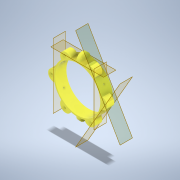
# Autodesk Inventor part: Connector
Saved by Autodesk Inventor 2021.2 (Build 252289000, 289)
## iProperties
Created: 2021-03-12
Part Number: Connector
Material: Generic
Document SubType Name: Modeling
Designer: Ryan
Density: 1 g/cm^3
Appearance: Smooth - Yellow
Author: Ryan
Autodesk Inventor part; units mm, degrees
ref_plane "XY Plane" through (0, 0, 0) normal (0, 0, 1) x (1, 0, 0)
sketch "Sketch1" plane through (0, 0, 0) normal (0, 0, 1) x (1, 0, 0)
  circle A0 centre (0, 0) radius 50.8
  circle A1 centre (0, 0) radius 53.975
  dimension "d0" = 101.6
  dimension "d1" = 107.95
  constraints: 2 centre point, 2 coincident
  measures "d0" diameter of A0
  measures "d1" diameter of A1
extrude "Extrusion1" add sketch "Sketch1" along normal blind 25.4
ref_plane "Work Plane1" through (38.1, 0, 0) normal (1, 0, 0) x (0, 1, 0)
ref_plane "Work Plane2" through (0, 53.975, 0) normal (0, 1, 0) x (-1, 0, 0)
sketch "Sketch3" plane through (0, 53.975, 0) normal (0, 1, 0) x (-1, 0, 0)
  line L0 (53.975, 0) -> (-53.975, 0) projected
  line L1 (3.175, 25.4) -> (-3.175, 25.4)
  line L2 (-3.175, 25.4) -> (-3.175, 0)
  line L3 (-3.175, 0) -> (3.175, 0)
  line L4 (3.175, 0) -> (3.175, 25.4)
  line L5 (3.175, 25.4) -> (-3.175, 0) construction
  line L6 (-3.175, 25.4) -> (3.175, 0) construction
  line L7 (53.975, 25.4) -> (-53.975, 25.4) projected
  point P0 (0, 0)
  point P1 (0, 12.7)
  point P2 (3.175, 0)
  dimension "d11" = 6.35
  dimension "d12" = 0
  constraints: 12 end point, 2 midpoint, 2 parallel, 1 horizontal, 1 perpendicular, 1 point on line
  measures "d11" distance of L3.end L2.end
  measures "d12" distance between parallel lines of L7 L1
extrude "Extrusion3" add sketch "Sketch3" along normal blind 12.7
fillet "Fillet1" radius 12.7 2 edges at (0, 66.675, 25.4) (0, 66.675, 0)
sketch "Sketch4" plane through (3.175, 53.975, 25.4) normal (1, 0, 0) x (0, 0, -1)
  circle A0 centre (6.35, 5.08) radius 1.5875
  line L0 (-5.08, 0) -> (30.48, 0) projected
  line L1 (0, 0) -> (0, -107.95) projected
  circle A1 centre (19.05, 5.08) radius 1.5875
  line L2 (25.4, 0) -> (25.4, -107.95) projected
  point P0 (25.4, -53.975)
  dimension "d16" = 3.175
  dimension "d17" = 5.08
  dimension "d40" = 6.35
  dimension "d41" = 3.175
  dimension "d42" = 6.35
  dimension "d43" = 5.08
  constraints: 2 centre point
  measures "d16" diameter of A0
  measures "d17" distance from line of L0 A0.centre
  measures "d40" horizontal distance of A0.centre L1.start
  measures "d41" diameter of A1
  measures "d42" horizontal distance of L2.start A1.centre
  measures "d43" distance from line of L0 A1.centre
extrude "Extrusion4" cut sketch "Sketch4" against normal blind 12.7
pattern_circular "Circular Pattern2" count 2 over 360 about axis through (0, 0, 0) along (0, 0, 1) of "Extrusion4", "Fillet1", "Extrusion3"
ref_plane "Work Plane3" through (-53.975, 0, 0) normal (1, 0, 0) x (0, 1, 0)
sketch "Sketch5" plane through (-53.975, 0, 0) normal (1, 0, 0) x (0, 1, 0)
  line L0 (-12.7, 9.525) -> (12.7, 9.525)
  line L1 (12.7, 9.525) -> (12.7, 15.875)
  line L2 (12.7, 15.875) -> (-12.7, 15.875)
  line L3 (-12.7, 15.875) -> (-12.7, 9.525)
  line L4 (-12.7, 9.525) -> (12.7, 15.875) construction
  line L5 (12.7, 9.525) -> (-12.7, 15.875) construction
  line L6 (53.975, 25.4) -> (-53.975, 25.4) projected
  line L7 (12.7, 15.875) -> (-12.7, 15.875)
  line L8 (-12.7, 15.875) -> (-12.7, 25.4)
  line L9 (-12.7, 25.4) -> (12.7, 25.4)
  line L10 (12.7, 25.4) -> (12.7, 15.875)
  point P0 (0, 0)
  point P1 (0, 12.7)
  point P2 (12.7, 25.4)
  dimension "d24" = 25.4
  dimension "d25" = 6.35
  dimension "d26" = 12.7
  dimension "d27" = 0
  constraints: 20 end point, 4 parallel, 2 horizontal, 2 midpoint, 2 perpendicular, 1 point on line
  measures "d24" distance of L2.end L1.end
  measures "d25" distance of L1.end L0.end
  measures "d26" distance of point (0, 12.7) point (0, 0)
  measures "d27" horizontal distance of point (0, 12.7) point (0, 0)
extrude "Extrusion8" add sketch "Sketch5" along normal blind 2.54
sketch "Sketch8" plane through (-53.975, 0, 0) normal (-1, 0, 0) x (0, 0, 1)
  line L0 (9.525, 0) -> (9.525, -12.7) projected
  line L1 (9.525, 12.7) -> (25.4, 12.7) projected
  line L2 (9.525, -12.7) -> (25.4, -12.7)
  line L3 (25.4, -12.7) -> (25.4, 12.7)
  line L4 (25.4, 12.7) -> (9.525, 12.7)
  line L5 (9.525, 12.7) -> (9.525, -12.7)
  point P0 (0, 0)
  constraints: 8 end point, 2 parallel, 1 horizontal, 1 perpendicular
extrude "Extrusion9" add sketch "Sketch8" along normal blind 12.7
fillet "Fillet3" radius 12.7 2 edges at (-66.675, 12.7, 17.4625) (-66.675, -12.7, 17.4625)
sketch "Sketch9" plane through (0, 0, 9.525) normal (0, 0, -1) x (-1, 0, 0)
  circle A0 centre (59.055, 0) radius 3.175
  line L0 (53.975, -93.345) -> (53.975, 93.345) projected
  point P0 (0, 0)
  dimension "d54" = 5.08
  dimension "d55" = 6.35
  constraints: 1 centre point
  measures "d54" distance from line of L0 A0.centre
  measures "d55" diameter of A0
extrude "Extrusion10" cut sketch "Sketch9" against normal through all
pattern_circular "Circular Pattern4" count 6 over 360 about axis through (0, 0, 0) along (0, 0, 1) of "Extrusion8", "Extrusion9", "Fillet3", "Extrusion10"
sketch "Sketch10" plane through (0, 53.975, 0) normal (0, 1, 0) x (-1, 0, 0)
  line L0 (3.175, 25.4) -> (3.175, 0) projected
  line L1 (-3.175, 0) -> (-3.175, 25.4) projected
  line L2 (3.175, 0) -> (-3.175, 0)
  line L3 (-3.175, 0) -> (-3.175, 25.4)
  line L4 (-3.175, 25.4) -> (3.175, 25.4)
  line L5 (3.175, 25.4) -> (3.175, 0)
  point P0 (0, 0)
  constraints: 8 end point, 2 parallel, 1 horizontal, 1 perpendicular
extrude "Extrusion11" add sketch "Sketch10" against normal blind 2.54
mirror "Mirror1" about plane through (0, 0, 0) normal (0, 1, 0) of "Extrusion11"
ref_plane "Work Plane4" through (46.7437, -26.9875, 0) normal (0.8660254, -0.5, 0) x (0.5, 0.8660254, 0)
sketch "Sketch11" plane through (46.7437, -26.9875, 0) normal (0.8660254, -0.5, 0) x (0.5, 0.8660254, 0)
  line L0 (12.5159, 12.7) -> (5.3749, 12.7)
  line L1 (53.975, 0) -> (-45.0753, 0) projected
  circle A0 centre (0, 12.7) radius 1.5875
  point P0 (0, 0)
  point P1 (48.2503, 0)
  dimension "d63" = 12.7
  dimension "d64" = 3.175
  constraints: 2 end point, 1 centre point, 1 horizontal
  measures "d63" distance between parallel lines of L1 L0
  measures "d64" diameter of A0
sketch "Sketch12" plane through (46.7437, -26.9875, 0) normal (0.8660254, -0.5, 0) x (0.5, 0.8660254, 0)
  line L0 (12.3111, 12.7) -> (5.5666, 12.7)
  line L1 (53.975, 0) -> (-45.0753, 0) projected
  circle A0 centre (0, 12.7) radius 6.35
  point P0 (0, 0)
  point P1 (48.2503, 0)
  dimension "d67" = 12.7
  dimension "d68" = 12.7
  constraints: 2 end point, 2 vertical alignment, 1 centre point, 1 horizontal
  measures "d67" distance between parallel lines of L1 L0
  measures "d68" diameter of A0
extrude "Extrusion13" add sketch "Sketch12" against normal blind 2.54
extrude "Extrusion14" cut sketch "Sketch11" along normal mid plane 25.4
pattern_circular "Circular Pattern5" count 2 over 360 about axis through (0, 0, 0) along (0, 0, 1) of "Extrusion13", "Extrusion14"
ref_plane "Work Plane6" through (46.7437, 26.9875, 0) normal (-0.8660254, -0.5, 0) x (0.5, -0.8660254, 0)
sketch "Sketch13" plane through (46.7437, 26.9875, 0) normal (-0.8660254, -0.5, 0) x (0.5, -0.8660254, 0)
  line L0 (-12.4208, 12.7) -> (-5.6891, 12.7)
  line L1 (53.975, 0) -> (-45.0753, 0) projected
  circle A0 centre (0, 12.7) radius 6.35
  point P0 (0, 0)
  point P1 (48.2503, 0)
  dimension "d76" = 12.7
  dimension "d77" = 12.7
  constraints: 2 end point, 1 centre point, 1 horizontal
  measures "d76" distance between parallel lines of L1 L0
  measures "d77" diameter of A0
extrude "Extrusion15" add sketch "Sketch13" along normal blind 2.54
sketch "Sketch14" plane through (46.7437, 26.9875, 0) normal (-0.8660254, -0.5, 0) x (0.5, -0.8660254, 0)
  line L0 (-13.2742, 12.7) -> (-9.3648, 12.7)
  line L1 (53.975, 0) -> (-45.0753, 0) projected
  circle A0 centre (0, 12.7) radius 1.5875
  point P0 (0, 0)
  point P1 (48.2503, 0)
  dimension "d80" = 12.7
  dimension "d81" = 3.175
  constraints: 2 end point, 1 centre point, 1 horizontal
  measures "d80" distance between parallel lines of L1 L0
  measures "d81" diameter of A0
extrude "Extrusion16" cut sketch "Sketch14" against normal mid plane 25.4
pattern_circular "Circular Pattern6" count 2 over 360 about axis through (0, 0, 0) along (0, 0, 1) of "Extrusion15", "Extrusion16"
body "Solid1"
